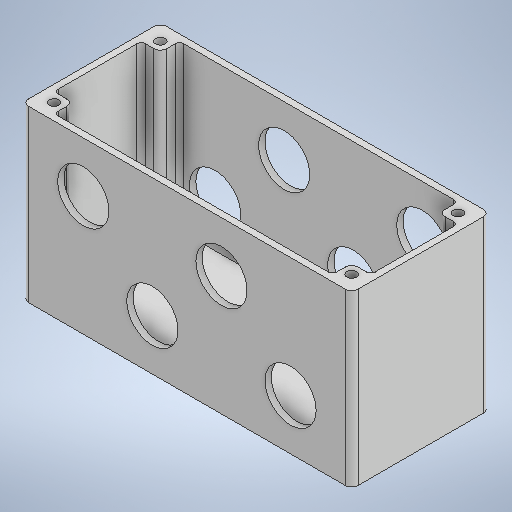
# Autodesk Inventor part: arcade_box_iteration3
Saved by Autodesk Inventor 2025.2 (Build 292293000, 293)
## iProperties
Created: 2025-03-25
Part Number: arcade_box_iteration3
Material: Generic
Document SubType Name: Modeling
Designer: osmon
Density: 1 g/cm^3
Appearance: Default
Author: osmon
Autodesk Inventor part; units mm, degrees
ref_plane "YZ Plane" through (0, 0, 0) normal (1, 0, 0) x (0, 1, 0)
ref_plane "XZ Plane" through (0, 0, 0) normal (0, 1, 0) x (-1, 0, 0)
ref_plane "XY Plane" through (0, 0, 0) normal (0, 0, 1) x (1, 0, 0)
sketch "Sketch1" plane through (0, 0, 0) normal (0, 1, 0) x (-1, 0, 0)
  line L0 (0, 0) -> (-155, 0)
  line L1 (-155, 0) -> (-155, -65)
  line L2 (-155, -65) -> (0, -65)
  line L3 (0, -65) -> (0, 0)
  dimension "d0" = 155
  dimension "d1" = 65
  constraints: 8 end point, 2 parallel, 1 horizontal, 1 perpendicular
  measures "d0" distance of L2.end L1.end
  measures "d1" distance of L1.end L0.end
extrude "Extrusion1" add sketch "Sketch1" along normal blind 80
sketch "Sketch2" plane through (0, 80, 0) normal (0, 1, 0) x (1, 0, 0)
  line L0 (155, 0) -> (155, 65) projected
  line L1 (155, 65) -> (0, 65) projected
  line L2 (0, 65) -> (0, 0) projected
  line L3 (0, 0) -> (155, 0) projected
  line L4 (3, 62) -> (152, 62)
  line L5 (152, 62) -> (152, 3)
  line L6 (152, 3) -> (3, 3)
  line L7 (3, 3) -> (3, 62)
  dimension "d4" = 3
  constraints: 8 end point, 3 other
  measures "d4" distance between parallel lines of L1 L4
extrude "Extrusion2" cut sketch "Sketch2" against normal blind 77 contours L4 L5 L6 L7
sketch "Sketch3" plane through (0, 0, 0) normal (0, 0, 1) x (1, 0, 0)
  circle A0 centre (28.75, 56.25) radius 12
  circle A1 centre (61.25, 23.75) radius 12
  circle A2 centre (93.75, 56.25) radius 12
  circle A3 centre (126.25, 23.75) radius 12
  point P0 (0, 0)
  dimension "d7" = 24
  dimension "d8" = 24
  dimension "d9" = 24
  dimension "d10" = 24
  constraints: 4 centre point
  measures "d7" diameter of A0
  measures "d8" diameter of A1
  measures "d9" diameter of A2
  measures "d10" diameter of A3
extrude "Extrusion3" cut sketch "Sketch3" against normal blind 3
sketch "Sketch4" plane through (155, 0, -65) normal (0, 0, -1) x (-1, 0, 0)
  circle A0 centre (28.75, 56.25) radius 12
  circle A1 centre (61.25, 23.75) radius 12
  circle A2 centre (93.75, 56.25) radius 12
  circle A3 centre (126.25, 23.75) radius 12
  point P0 (155, 0)
  dimension "d13" = 24
  dimension "d14" = 24
  dimension "d15" = 24
  dimension "d16" = 24
  constraints: 4 centre point
  measures "d13" diameter of A0
  measures "d14" diameter of A1
  measures "d15" diameter of A2
  measures "d16" diameter of A3
extrude "Extrusion4" cut sketch "Sketch4" against normal blind 3
sketch "Sketch5" plane through (0, 3, 0) normal (0, 1, 0) x (1, 0, 0)
  line L0 (152, 3) -> (3, 3) projected
  line L1 (152, 62) -> (152, 3) projected
  line L2 (3, 62) -> (152, 62) projected
  line L3 (3, 3) -> (3, 62) projected
  line L4 (3, 62) -> (12, 62)
  line L5 (12, 62) -> (12, 53)
  line L6 (12, 53) -> (3, 53)
  line L7 (3, 53) -> (3, 62)
  point P0 (0, 0)
  point P1 (3, 57.5)
  point P2 (3, 53)
  dimension "d19" = 9
  dimension "d20" = 9
  dimension "d21" = 0
  dimension "d22" = 0
  constraints: 8 end point, 2 parallel, 1 horizontal, 1 midpoint, 1 perpendicular
  measures "d19" distance of L5.end L6.end
  measures "d20" distance of L4.end L5.end
  measures "d21" distance between parallel lines of L2 L4
  measures "d22" distance from line of L3 point (3, 57.5)
extrude "Extrusion5" add sketch "Sketch5" along normal blind 77 contours L3 L2 L5 L6
fillet "Fillet1" radius 3 4 edges at (0, 40, 0) (0, 40, -65) (155, 40, -65) (155, 40, 0)
sketch "Sketch8" plane through (0, 80, 0) normal (0, 1, 0) x (1, 0, 0)
  circle A0 centre (7.5, 57.5) radius 2.25
  arc A1 (152, 0) -> (155, 3) centre (152, 3) ccw projected
  line L0 (155, 3) -> (155, 62) projected
  arc A2 (155, 62) -> (152, 65) centre (152, 62) ccw projected
  line L1 (152, 65) -> (3, 65) projected
  arc A3 (3, 65) -> (0, 62) centre (3, 62) ccw projected
  line L2 (0, 62) -> (0, 3) projected
  arc A4 (0, 3) -> (3, 0) centre (3, 3) ccw projected
  line L3 (3, 0) -> (152, 0) projected
  line L4 (3, 3) -> (3, 53) projected
  line L5 (3, 53) -> (12, 53) projected
  line L6 (12, 53) -> (12, 62) projected
  line L7 (12, 62) -> (152, 62) projected
  line L8 (152, 62) -> (152, 3) projected
  line L9 (152, 3) -> (3, 3) projected
  point P0 (0, 0)
  dimension "d45" = 4.5
  dimension "d46" = 4.5
  dimension "d47" = 4.5
  constraints: 1 centre point
  measures "d45" diameter of A0
  measures "d46" distance from line of L6 A0.centre
  measures "d47" distance from line of L5 A0.centre
extrude "Extrusion8" cut sketch "Sketch8" against normal blind 4.5 contours A0
sketch "Sketch9" plane through (7.5, 75.5, -57.5) normal (0, 1, 0) x (1, 0, 0)
  circle A0 centre (0, 0) radius 2.25 projected
  circle A1 centre (0, 0) radius 1.6
  point P0 (-7.5, -57.5)
  dimension "d50" = 3.2
  constraints: 1 centre point, 1 coincident
  measures "d50" diameter of A1
extrude "Extrusion9" cut sketch "Sketch9" against normal blind 2.5 contours A1
pattern_linear "Rectangular Pattern2" count 2 spacing 140 along (1, 0, 0) count 2 spacing -50 along (0, 0, -1) of "Extrusion5", "Extrusion8", "Extrusion9"
fillet "Fillet4" radius 3 4 edges at (12, 41.5, -53) (12, 41.5, -12) (143, 41.5, -53) (143, 41.5, -12)
fillet "Fillet5" radius 2 8 edges at (3, 41.5, -53) (12, 41.5, -62) (3, 41.5, -12) (12, 41.5, -3) (152, 41.5, -53) (143, 41.5, -62) (152, 41.5, -12) (143, 41.5, -3)
body "Solid1"
